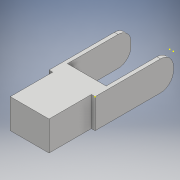
# Autodesk Inventor part: CRANEJ3
Saved by Autodesk Inventor 2017 (Build 210142000, 142)
## iProperties
Part Number: CRANEJ3
Material: 一般
Document SubType Name: Modeling
Designer: rsdlab
Density: 1 g/cm^3
Appearance: 既定
Author: rsdlab
Autodesk Inventor part; units mm, degrees
ref_plane "YZ Plane" through (0, 0, 0) normal (1, 0, 0) x (0, 1, 0)
ref_plane "XZ Plane" through (0, 0, 0) normal (0, 1, 0) x (-1, 0, 0)
ref_plane "XY Plane" through (0, 0, 0) normal (0, 0, 1) x (1, 0, 0)
sketch "スケッチ1" plane through (0, 0, 0) normal (0, 1, 0) x (-1, 0, 0)
  line L0 (0, 0) -> (0.04, 0)
  line L1 (0.04, 0) -> (0.04, -0.32)
  line L2 (0.04, -0.32) -> (0, -0.32)
  line L3 (0, -0.32) -> (0, 0)
  line L4 (0.46, 0) -> (0.5, 0)
  line L5 (0.5, 0) -> (0.5, -0.32)
  line L6 (0.5, -0.32) -> (0.46, -0.32)
  line L7 (0.46, -0.32) -> (0.46, 0)
  dimension "d2" = 0.04
  dimension "d3" = 0.32
  dimension "d8" = 0.04
  dimension "d9" = 0.32
  constraints: 16 end point, 4 parallel, 2 horizontal, 2 perpendicular
  measures "d2" distance of L1.end L2.end
  measures "d3" distance of L0.end L1.end
  measures "d8" distance of L5.end L6.end
  measures "d9" distance of L4.end L5.end
extrude "押し出し1" add sketch "スケッチ1" against normal blind 0.69
sketch "スケッチ2" plane through (0, -0.69, 0) normal (0, -1, 0) x (1, 0, 0)
  line L0 (-0.5, -0.32) -> (-0.46, -0.32) projected
  line L1 (0, 0) -> (-0.5, 0)
  line L2 (-0.5, 0) -> (-0.5, -0.32)
  line L3 (-0.5, -0.32) -> (0, -0.32)
  line L4 (0, -0.32) -> (0, 0)
  constraints: 8 end point, 2 parallel, 1 horizontal, 1 perpendicular
extrude "押し出し2" add sketch "スケッチ2" along normal blind 0.16
sketch "スケッチ3" plane through (0, -0.85, 0) normal (0, -1, 0) x (1, 0, 0)
  point P0 (0, 0)
sketch "スケッチ4" plane through (0, -0.85, 0) normal (0, -1, 0) x (1, 0, 0)
  line L0 (-0.04, 0) -> (-0.04, -0.32) projected
  line L1 (-0.46, -0.32) -> (-0.04, -0.32) projected
  line L2 (-0.04, 0) -> (-0.46, 0)
  line L3 (-0.46, 0) -> (-0.46, -0.32)
  line L4 (-0.46, -0.32) -> (-0.04, -0.32)
  line L5 (-0.04, -0.32) -> (-0.04, 0)
  point P0 (0, 0)
  dimension "d12" = 0.42
  constraints: 8 end point, 2 parallel, 1 horizontal, 1 perpendicular
  measures "d12" distance of L4.end L1.start
extrude "押し出し3" add sketch "スケッチ4" along normal blind 0.46
fillet "フィレット1" radius 0.14 4 edges at (-0.02, 0, 0) (-0.02, 0, -0.32) (-0.48, 0, 0) (-0.48, 0, -0.32)
sketch "スケッチ5" plane through (0, -0.85, 0) normal (1, 0, 0) x (0, 0, -1)
  point P0 (0, 0.85)
sketch "スケッチ6" plane through (-0.04, -0.85, 0) normal (1, 0, 0) x (0, 0, -1)
  point P0 (0, 0.85)
